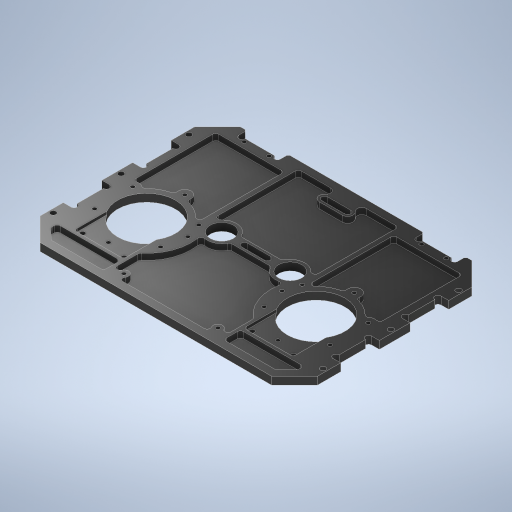
# Autodesk Inventor part: TorsoPelvisLowerFrame
Saved by Autodesk Inventor 2024.2 (Build 282272000, 272)
## iProperties
Created: 2024-01-05
Part Number: TorsoPelvisLowerFrame
Material: Aluminum 7075
Document SubType Name: Modeling
Designer: Masato Kubotera
Density: 2.81 g/cm^3
Appearance: Glossy - Black
Mass: 131.437 g
Surface Area: 496.225 cm^2
Volume: 46.7747 cm^3
Vendor: meviy
Author: Masato Kubotera
Autodesk Inventor part; units mm, degrees
ref_plane "YZ Plane" through (0, 0, 0) normal (1, 0, 0) x (0, 1, 0)
ref_plane "XZ Plane" through (0, 0, 0) normal (0, 1, 0) x (-1, 0, 0)
sketch "Sketch1" plane through (0, 0, 0) normal (0, 0, 1) x (1, 0, 0)
  line L0 (-65, -90) -> (65, -90)
  line L1 (65, -90) -> (65, 90)
  line L2 (65, 90) -> (-65, 90) construction
  line L3 (-65, 90) -> (-65, -90)
  line L4 (65, -90) -> (-65, 90) construction
  line L5 (-65, 0) -> (65, 0)
  line L6 (0, -90) -> (0, 90) construction
  circle A0 centre (16, 55) radius 18.75
  line L7 (16, 55) -> (40.75, 55) construction
  circle A1 centre (16, 55) radius 29 construction
  line L8 (4, 39) -> (47, 39) construction
  line L9 (47, 39) -> (47, 71) construction
  line L10 (47, 71) -> (4, 71) construction
  line L11 (4, 71) -> (4, 39) construction
  line L12 (4, 39) -> (47, 71) construction
  line L13 (47, 39) -> (4, 71) construction
  line L14 (17, 41.5) -> (44, 41.5) construction
  line L15 (44, 41.5) -> (44, 68.5) construction
  line L16 (44, 68.5) -> (17, 68.5) construction
  line L17 (17, 68.5) -> (17, 41.5) construction
  line L18 (17, 41.5) -> (44, 68.5) construction
  line L19 (44, 41.5) -> (17, 68.5) construction
  line L20 (10, 90) -> (10, 85) construction
  line L21 (35, 85) -> (35, 90) construction
  line L22 (65, 87.5) -> (-65, 87.5) construction
  line L23 (9.95, 90) -> (9.95, 85)
  line L24 (35.05, 85) -> (35.05, 90)
  line L25 (22.5, 85) -> (22.5, 90) construction
  line L26 (9.95, 85) -> (35.05, 85)
  line L27 (-10, 90) -> (-10, 85) construction
  line L28 (-35, 85) -> (-35, 90) construction
  line L29 (-9.95, 90) -> (-9.95, 85)
  line L30 (-35.05, 85) -> (-35.05, 90)
  line L31 (-22.5, 85) -> (-22.5, 90) construction
  line L32 (-9.95, 85) -> (-35.05, 85)
  arc A2 (31.05, 85) -> (35.05, 85) centre (33.05, 85) ccw
  arc A3 (9.95, 85) -> (13.95, 85) centre (11.95, 85) ccw
  arc A4 (-35.05, 85) -> (-31.05, 85) centre (-33.05, 85) ccw
  arc A5 (-13.95, 85) -> (-9.95, 85) centre (-11.95, 85) ccw
  line L33 (-65, 90) -> (-35.05, 90)
  line L34 (-10, 90) -> (9.95, 90)
  line L35 (35.05, 90) -> (65, 90)
  line L36 (25.6933, 38.95) -> (47, 38.95)
  line L37 (47, 38.95) -> (47, 71.05)
  line L38 (47, 71.05) -> (25.6933, 71.05)
  line L39 (9.5, -37.5) -> (59.5, -37.5) construction
  line L40 (59.5, -37.5) -> (59.5, 37.5) construction
  line L41 (59.5, 37.5) -> (9.5, 37.5) construction
  line L42 (9.5, 37.5) -> (9.5, -37.5) construction
  line L43 (9.5, -37.5) -> (59.5, 37.5) construction
  line L44 (59.5, -37.5) -> (9.5, 37.5) construction
  line L45 (13.75, -30.5) -> (55.25, -30.5) construction
  line L46 (55.25, -30.5) -> (55.25, 30.5) construction
  line L47 (55.25, 30.5) -> (13.75, 30.5) construction
  line L48 (13.75, 30.5) -> (13.75, -30.5) construction
  line L49 (13.75, -30.5) -> (55.25, 30.5) construction
  line L50 (55.25, -30.5) -> (13.75, 30.5) construction
  circle A6 centre (0, 22.1938) radius 7.5
  line L51 (60, 0) -> (60, 26.3242)
  line L52 (53.0706, 37) -> (38.7376, 37)
  arc A7 (53.9423, 33.2) -> (56.9, 27.9945) centre (55.25, 30.5) ccw
  arc A8 (3.5, 13.362) -> (8.1445, 27.0842) centre (0, 22.1938) ccw
  line L53 (3.5, 13.362) -> (3.5, 0)
  line L54 (49, 38.95) -> (60, 38.95)
  line L55 (60, 38.95) -> (60, 72.9289)
  line L56 (49, 80) -> (49, 38.95)
  line L57 (-60, 0) -> (-60, 32.5463)
  line L58 (-53.9, 35.5463) -> (-53.9, 78)
  arc A9 (-6.53, 29.0937) -> (-3.5, 13.362) centre (0, 22.1938) ccw
  arc A10 (-6.2374, 58.4277) -> (-6.2374, 51.5723) centre (-8.75, 55) ccw
  arc A11 (-6.2374, 51.5723) -> (0.21, 38.9711) centre (16, 55) ccw
  arc A12 (1.9128, 72.5443) -> (-6.2374, 58.4277) centre (16, 55) ccw
  line L59 (-3.5, 13.362) -> (-3.5, 0)
  line L60 (65, 75) -> (50, 90)
  line L61 (-65, 75) -> (-50, 90)
  line L62 (-50, -70) -> (-2, -70) construction
  line L63 (-2, -70) -> (-2, 70) construction
  line L64 (-2, 70) -> (-50, 70) construction
  line L65 (-50, 70) -> (-50, -70) construction
  line L66 (-50, -70) -> (-2, 70) construction
  line L67 (-2, -70) -> (-50, 70) construction
  line L68 (-26, -70) -> (-26, 70) construction
  arc A13 (-1.1936, 35.5463) -> (0.21, 38.9711) centre (-1.1936, 37.5463) ccw
  line L69 (-1.1936, 35.5463) -> (-53.9, 35.5463)
  line L70 (-60, 32.5463) -> (-7.9047, 32.5463)
  arc A14 (1.3126, 80) -> (1.9128, 72.5443) centre (3.625, 76.4341) ccw
  line L71 (-51.9, 80) -> (1.3126, 80)
  arc A15 (-50, 7.5) -> (-54, 7.5) centre (-52, 7.5) ccw
  line L72 (-50, 7.5) -> (-50, 0)
  line L73 (-54, 7.5) -> (-54, 0)
  arc A16 (2, 7.5) -> (-2, 7.5) centre (0, 7.5) ccw
  line L74 (-2, 7.5) -> (-2, 0)
  line L75 (2, 7.5) -> (2, 0)
  arc A17 (-6.53, 29.0937) -> (-7.9047, 32.5463) centre (-7.9047, 30.5463) ccw
  line L76 (60, 72.9289) -> (52.9289, 80)
  line L77 (52.9289, 80) -> (49, 80)
  circle A18 centre (3.625, 33.5659) radius 4.25 construction
  arc A19 (8.1445, 27.0842) -> (38.7376, 37) centre (16, 55) ccw
  arc A20 (60, 26.3242) -> (56.9, 27.9945) centre (58, 26.3242) ccw
  arc A21 (53.9423, 33.2) -> (53.0706, 37) centre (53.0706, 35) ccw
  arc A22 (-48.5, 7.5) -> (-55.5, 7.5) centre (-52, 7.5) ccw
  line L78 (-48.5, 0) -> (-48.5, 7.5)
  line L79 (-55.5, 0) -> (-55.5, 7.5)
  arc A23 (-60, 11.6533) -> (-54.6923, 9.7364) centre (-57, 11.6533) ccw
  line L80 (34.5, -38.1517) -> (34.5, 37.5) construction
  line L81 (-65.8, 45) -> (-53.9, 45) construction
  line L82 (-53.9, 45) -> (-53.9, 70) construction
  line L83 (-53.9, 70) -> (-65.8, 70) construction
  line L84 (-65.8, 70) -> (-65.8, 45) construction
  line L85 (-65.8, 45) -> (-53.9, 70) construction
  line L86 (-53.9, 45) -> (-65.8, 70) construction
  line L87 (-65.8, 57.5) -> (-53.9, 57.5) construction
  line L88 (-57.9, 45) -> (-57.9, 70) construction
  line L89 (-65, 44) -> (-59.9, 44)
  line L90 (-59.9, 44) -> (-59.9, 71)
  line L91 (-59.9, 71) -> (-65, 71)
  arc A24 (-59.9, 44) -> (-59.9, 48) centre (-59.9, 46) ccw
  arc A25 (-59.9, 67) -> (-59.9, 71) centre (-59.9, 69) ccw
  line L92 (-60, 45) -> (-60, 70) construction
  arc A26 (-51.9, 80) -> (-53.9, 78) centre (-51.9, 78) ccw
  point P0 (0, 0)
  point P1 (28.375, 76.4341)
  point P2 (28.375, 33.5659)
  point P3 (25.5, 55)
  point P4 (30.5, 55)
  point P5 (44, 87.5)
  point P6 (0, 87.5)
  point P7 (-44, 87.5)
  point P8 (-9.95, 90)
  point P9 (-35.05, 90)
  point P10 (-31.05, 85)
  point P11 (13.95, 85)
  point P12 (-13.95, 85)
  point P13 (49.625, 0)
  point P14 (-27.05, 85)
  point P15 (13.95, 85)
  point P16 (-13.95, 85)
  point P17 (-9.95, 90)
  point P18 (17, 55)
  point P19 (34.5, 0)
  point P20 (-3.5, 0)
  point P21 (-50, 90)
  point P22 (-26, 0)
  point P23 (8, 0)
  point P24 (-52.9289, 80)
  point P25 (2, 0)
  point P26 (-50, 0)
  point P27 (-2, 0)
  point P28 (-1.5, 10)
  point P29 (60, 72.9289)
  point P30 (-55.5, 0)
  point P31 (-48.5, 0)
  point P32 (-59.85, 57.5)
  point P33 (-57.9, 49.5)
  point P34 (-57.9, 65.5)
  point P35 (-59.9, 67)
  dimension "d0" = 130
  dimension "d1" = 180
  dimension "d2" = 37.5
  dimension "d6" = 360
  dimension "d8" = 58
  dimension "d9" = 49.5
  dimension "d10" = 43
  dimension "d11" = 32
  dimension "d12" = 27
  dimension "d13" = 27
  dimension "d21" = 5
  dimension "d22" = 0.05
  dimension "d23" = 20
  dimension "d25" = 25
  dimension "d52" = 2
  dimension "d151" = 110
  dimension "d154" = 0.05
  dimension "d156" = 16
  dimension "d158" = 9.5
  dimension "d159" = 8.5
  dimension "d160" = 50
  dimension "d161" = 75
  dimension "d163" = 7
  dimension "d165" = 15
  dimension "d166" = 29.3875
  dimension "d167" = 5
  dimension "d168" = 6
  dimension "d172" = 2
  dimension "d174" = 2
  dimension "d175" = 2
  dimension "d176" = 9
  dimension "d184" = 15
  dimension "d186" = 45
  dimension "d187" = 48
  dimension "d188" = 140
  dimension "d195" = 3
  dimension "d202" = 5
  dimension "d206" = 4
  dimension "d207" = 15
  dimension "d208" = 1.5
  dimension "d209" = 41.5
  dimension "d211" = 45
  dimension "d214" = 2
  dimension "d216" = 3
  dimension "d217" = 11.9
  dimension "d218" = 25
  dimension "d219" = 16
  dimension "d220" = 0.8
  dimension "d221" = 1
  dimension "d223" = 5
  dimension "d224" = 4
  dimension "d225" = 5
  dimension "d227" = 5
  dimension "d228" = 0.1
  dimension "d229" = 5
  dimension "d230" = 115
  constraints: 188 end point, 51 point on circle, 34 point on line, 33 symmetric about line, 27 centre point, 26 midpoint, 20 tangent, 18 horizontal, 18 vertical, 16 parallel, 15 coincident, 8 equal radius, 7 collinear, 7 perpendicular, 1 concentric, 27 other
  measures "d0" distance of L2.end L1.end
  measures "d1" distance of L1.end L0.end
  measures "d2" diameter of A0
  measures "d8" diameter of A1
  measures "d9" distance of point (40.75, 55) point (-8.75, 55)
  measures "d10" distance of L10.end L9.end
  measures "d11" distance of L9.end L8.end
  measures "d12" distance of L16.end L15.end
  measures "d13" distance of L15.end L14.end
  measures "d21" distance of L21.start L21.end
  measures "d22" distance between parallel lines of L24 L21
  measures "d23" distance between parallel lines of L20 L27
  measures "d25" distance between parallel lines of L21 L20
  measures "d52" radius of A2
  measures "d154" distance between parallel lines of L36 L8
  measures "d156" distance from line of L7.start L6
  measures "d158" distance of point (25.5, 55) A1.centre
  measures "d159" distance of point (17, 55) point (25.5, 55)
  measures "d160" distance of L41.end L40.end
  measures "d161" distance of L40.end L39.end
  measures "d163" vertical distance of L40.end L46.end
  measures "d165" diameter of A6
  measures "d167" distance between parallel lines of L1 L51
  measures "d168" diameter of A7
  measures "d172" radial gap between concentric circles of A8 A6
  measures "d174" distance between parallel lines of L52 L8
  measures "d175" distance between parallel lines of L56 L37
  measures "d176" distance from line of point (44, 87.5) L21
  measures "d184" distance from line of L60.end L21
  measures "d186" angle of L60 L2
  measures "d187" distance of L64.end L63.end
  measures "d188" distance of L63.end L62.end
  measures "d195" distance between parallel lines of L69 L70
  measures "d202" distance between parallel lines of L71 L32
  measures "d206" diameter of A15
  measures "d208" distance from line of L53.end L75
  measures "d209" distance of L45.start L45.end
  measures "d211" diameter of A11
  measures "d214" radius of A13
  measures "d216" radius of A23
  measures "d217" distance of L83.end L82.end
  measures "d218" distance of L82.end L81.end
  measures "d219" distance of point (-57.9, 65.5) point (-57.9, 49.5)
  measures "d220" distance between parallel lines of L3 L84
  measures "d221" distance between parallel lines of L91 L83
  measures "d223" distance from line of L61.start L83
  measures "d224" distance between parallel lines of L88 L82
  measures "d225" distance between parallel lines of L92 L3
  measures "d227" distance between parallel lines of L57 L3
  measures "d228" distance between parallel lines of L90 L92
  measures "d229" distance between parallel lines of L60 L76
extrude "Extrusion1" add sketch "Sketch1" against normal blind 5 contours L3 L89 A24 L90 A25 L91 L61 L33 L30 A4 L32 A5 L29 L34 L23 A3 L26 A2 L24 L35 L60 L1 L5 L51 A20 A7 A21 L52 A19 A8 L53 L75 A16 L74 L59 A9 A17 L70 L57 | L57 A23 A22 L79 L5 | L5 L53 A8 A19 L52 A21 A7 A20 L51 | L79 A22 L78 L5 L72 A15 L73 | L57 L70 A17 A9 L59 L5 L78 A22 A23 | A0 L38 L37 L36 | L56 L77 L76 L55 L54 | L58 A26 L71 A14 A12 A10 A11 A13 L69
extrude "Extrusion2" cut sketch "Sketch1" against normal blind 2 contours A0 L38 L37 L36
extrude "Extrusion3" cut sketch "Sketch1" against normal blind 4 contours L5 L53 A8 A19 L52 A21 A7 A20 L51 | L57 L70 A17 A9 L59 L5 L78 A22 A23 | L73 A15 L72 L5 | L5 L74 A16 L75 | L56 L77 L76 L55 L54 | L58 A26 L71 A14 A12 A10 A11 A13 L69
hole "M3" at (28.375, 33.5659, 0) at (3.625, 33.5659, 0) at (40.75, 55, 0) at (28.375, 76.4341, 0) at (3.625, 76.4341, 0) at (-8.75, 55, 0) at (13.75, 30.5, 0) at (55.25, 30.5, 0) at (-57.9, 65.5, 0) at (-57.9, 49.5, 0) direction (0, 0, -1) diameter 2.459 end through all thread size "M3x0.5" class "6H" standard "ANSI Metric M Profile"
hole "Phi3.5" at (44, 87.5, 0) at (0, 87.5, 0) at (-44, 87.5, 0) direction (0, 0, -1) diameter 3.5 end through all
hole "Phi3.1" at (44, 41.5, 0) at (44, 68.5, 0) direction (0, 0, -1) diameter 3.1 end through all
fillet "R2" radius 2 19 edges at (47, 38.95, -1) (47, 71.05, -1) (3.5, 13.362, -2) (-6.53, 29.0937, -2) (-3.5, 13.362, -2) (-7.9047, 32.5463, -2) (-6.2374, 51.5723, -2) (-6.2374, 58.4277, -2) (1.9128, 72.5443, -2) (-60, 32.5463, -2) (1.3126, 80, -2) (60, 38.95, -2) (49, 38.95, -2) (49, 80, -2) (52.9289, 80, -2) (8.1445, 27.0842, -2) (38.7376, 37, -2) (-53.9, 35.5463, -2) (60, 72.9289, -2)
mirror "Mirror1" about plane through (65, 0, 0) normal (0, -1, 0)
ref_plane "Work Plane1" through (-26, 0, 0) normal (-1, 0, 0) x (0, 0, 1)
chamfer "C1" distance 1 angle 45 4 edges at (-65, 71, -2.5) (-65, 44, -2.5) (-65, -71, -2.5) (-65, -44, -2.5)
body "Solid1"
